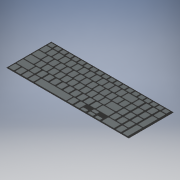
# Autodesk Inventor part: KEYBOARD
Saved by Autodesk Inventor 2017 (Build 210142000, 142)
## iProperties
Created: 2017-02-18
Part Number: KEYBOARD
Material: Generic
Document SubType Name: Modeling
Designer: Ali
Density: 1 g/cm^3
Appearance: Default
Author: Ali
Autodesk Inventor part; units mm, degrees
ref_plane "YZ Plane" through (0, 0, 0) normal (1, 0, 0) x (0, 1, 0)
ref_plane "XZ Plane" through (0, 0, 0) normal (0, 1, 0) x (-1, 0, 0)
ref_plane "XY Plane" through (0, 0, 0) normal (0, 0, 1) x (1, 0, 0)
sketch "Sketch1" plane through (0, 0, 0) normal (0, 1, 0) x (-1, 0, 0)
  line L0 (149.99, -109.99) -> (-149.99, -109.99)
  line L1 (-149.99, -109.99) -> (-149.99, 0)
  line L2 (-149.99, 0) -> (149.99, 0)
  line L3 (149.99, 0) -> (149.99, -109.99)
  dimension "d2" = 299.98
  dimension "d3" = 109.99
  constraints: 8 end point, 2 parallel, 1 horizontal, 1 perpendicular
  measures "d2" distance of L1.end L2.end
  measures "d3" distance of L0.end L1.end
extrude "KEYBOARD BASE" add sketch "Sketch1" along normal blind 0.01
sketch "Sketch2" plane through (0, 0.01, 0) normal (0, 1, 0) x (1, 0, 0)
  line L0 (-146.9909, 107.99) -> (-136.9909, 107.99)
  line L1 (-135.9909, 106.99) -> (-135.9909, 98.99)
  line L2 (-136.9909, 97.99) -> (-146.9909, 97.99)
  line L3 (-147.9909, 98.99) -> (-147.9909, 106.99)
  arc A0 (-146.9909, 107.99) -> (-147.9909, 106.99) centre (-146.9909, 106.99) ccw
  arc A1 (-135.9909, 106.99) -> (-136.9909, 107.99) centre (-136.9909, 106.99) ccw
  arc A2 (-136.9909, 97.99) -> (-135.9909, 98.99) centre (-136.9909, 98.99) ccw
  arc A3 (-147.9909, 98.99) -> (-146.9909, 97.99) centre (-146.9909, 98.99) ccw
  point P0 (0, 0)
  point P1 (-147.9909, 107.99)
  point P2 (-135.9909, 97.99)
  point P3 (-135.9909, 107.99)
  point P4 (-147.9909, 97.99)
  dimension "d9" = 10
  dimension "d10" = 12
  dimension "d150" = 1
  constraints: 8 end point, 8 point on circle, 8 point on line, 8 tangent, 4 centre point, 3 equal radius, 2 parallel, 1 horizontal, 1 perpendicular
  measures "d9" distance of point (-147.991, 97.99) point (-147.991, 107.99)
  measures "d10" distance of point (-147.991, 107.99) point (-135.991, 107.99)
  measures "d150" radius of A0
extrude "ESCAPE BUTTON" add sketch "Sketch2" along normal blind 0.3
pattern_linear "1ST ROW" count 20 spacing 14.75 along (1, 0, 0) of "ESCAPE BUTTON"
sketch "Sketch3" plane through (0, 0.01, 0) normal (0, 1, 0) x (1, 0, 0)
  line L0 (-145.9909, 95.99) -> (-136.4909, 95.99)
  line L1 (-134.4909, 93.99) -> (-134.4909, 80.79)
  line L2 (-136.4909, 78.79) -> (-145.9909, 78.79)
  line L3 (-147.9909, 80.79) -> (-147.9909, 93.99)
  arc A0 (-145.9909, 95.99) -> (-147.9909, 93.99) centre (-145.9909, 93.99) ccw
  arc A1 (-134.4909, 93.99) -> (-136.4909, 95.99) centre (-136.4909, 93.99) ccw
  arc A2 (-136.4909, 78.79) -> (-134.4909, 80.79) centre (-136.4909, 80.79) ccw
  arc A3 (-147.9909, 80.79) -> (-145.9909, 78.79) centre (-145.9909, 80.79) ccw
  point P0 (-147.9909, 95.99)
  point P1 (-134.4909, 78.79)
  point P2 (-134.4909, 95.99)
  point P3 (-147.9909, 78.79)
  dimension "d19" = 13.5
  dimension "d20" = 17.2
  dimension "d151" = 2
  constraints: 8 end point, 8 point on circle, 8 point on line, 8 tangent, 4 centre point, 3 equal radius, 2 parallel, 1 horizontal, 1 perpendicular
  measures "d19" distance of point (-147.991, 95.99) point (-134.491, 95.99)
  measures "d20" distance of point (-147.991, 78.79) point (-147.991, 95.99)
  measures "d151" radius of A0
extrude "2ND ROW" add sketch "Sketch3" along normal blind 0.3
pattern_linear "2ND ROW PATTERN" count 13 spacing 15.5 along (1, 0, 0) of "2ND ROW"
sketch "Sketch6" plane through (0, 0.01, 0) normal (0, 1, 0) x (1, 0, 0)
  line L0 (133.5089, 95.99) -> (143.0089, 95.99)
  line L1 (145.0089, 93.99) -> (145.0089, 80.79)
  line L2 (143.0089, 78.79) -> (133.5089, 78.79)
  line L3 (131.5089, 80.79) -> (131.5089, 93.99)
  arc A0 (133.5089, 95.99) -> (131.5089, 93.99) centre (133.5089, 93.99) ccw
  arc A1 (145.0089, 93.99) -> (143.0089, 95.99) centre (143.0089, 93.99) ccw
  arc A2 (143.0089, 78.79) -> (145.0089, 80.79) centre (143.0089, 80.79) ccw
  arc A3 (131.5089, 80.79) -> (133.5089, 78.79) centre (133.5089, 80.79) ccw
  point P0 (0, 0)
  point P1 (131.5089, 95.99)
  point P2 (145.0089, 78.79)
  point P3 (145.0089, 95.99)
  point P4 (131.5089, 78.79)
  dimension "d52" = 13.5
  dimension "d53" = 17.2
  dimension "d157" = 2
  constraints: 8 end point, 8 point on circle, 8 point on line, 8 tangent, 4 centre point, 3 equal radius, 2 parallel, 1 horizontal, 1 perpendicular
  measures "d52" distance of point (145.009, 78.79) point (131.509, 78.79)
  measures "d53" distance of point (145.009, 95.99) point (145.009, 78.79)
  measures "d157" radius of A0
sketch "Sketch4" plane through (0, 0.01, 0) normal (0, 1, 0) x (1, 0, 0)
  line L0 (55.5091, 95.99) -> (76.5091, 95.99)
  line L1 (78.5091, 93.99) -> (78.5091, 80.79)
  line L2 (76.5091, 78.79) -> (55.5091, 78.79)
  line L3 (53.5091, 80.79) -> (53.5091, 93.99)
  arc A0 (55.5091, 95.99) -> (53.5091, 93.99) centre (55.5091, 93.99) ccw
  arc A1 (78.5091, 93.99) -> (76.5091, 95.99) centre (76.5091, 93.99) ccw
  arc A2 (76.5091, 78.79) -> (78.5091, 80.79) centre (76.5091, 80.79) ccw
  arc A3 (53.5091, 80.79) -> (55.5091, 78.79) centre (55.5091, 80.79) ccw
  point P0 (53.5091, 95.99)
  point P1 (78.5091, 78.79)
  point P2 (78.5091, 95.99)
  point P3 (53.5091, 78.79)
  dimension "d31" = 25
  dimension "d32" = 17.2
  dimension "d156" = 2
  constraints: 8 end point, 8 point on circle, 8 point on line, 8 tangent, 4 centre point, 3 equal radius, 2 parallel, 1 horizontal, 1 perpendicular
  measures "d31" distance of point (78.509, 78.79) point (53.509, 78.79)
  measures "d32" distance of point (78.509, 95.99) point (78.509, 78.79)
  measures "d156" radius of A0
extrude "BACKSPACE BUTTON" add sketch "Sketch4" along normal blind 0.3
sketch "Sketch7" plane through (0, 0.01, 0) normal (0, 1, 0) x (1, 0, 0)
  line L0 (133.5098, 76.99) -> (143.0098, 76.99)
  line L1 (145.0098, 74.99) -> (145.0098, 42.79)
  line L2 (143.0098, 40.79) -> (133.5098, 40.79)
  line L3 (131.5098, 42.79) -> (131.5098, 74.99)
  arc A0 (133.5098, 76.99) -> (131.5098, 74.99) centre (133.5098, 74.99) ccw
  arc A1 (145.0098, 74.99) -> (143.0098, 76.99) centre (143.0098, 74.99) ccw
  arc A2 (143.0098, 40.79) -> (145.0098, 42.79) centre (143.0098, 42.79) ccw
  arc A3 (131.5098, 42.79) -> (133.5098, 40.79) centre (133.5098, 42.79) ccw
  point P0 (0, 0)
  point P1 (131.5098, 76.99)
  point P2 (145.0098, 40.79)
  point P3 (145.0098, 76.99)
  point P4 (131.5098, 40.79)
  dimension "d56" = 13.5
  dimension "d57" = 36.2
  dimension "d158" = 2
  constraints: 8 end point, 8 point on circle, 8 point on line, 8 tangent, 4 centre point, 3 equal radius, 2 parallel, 1 horizontal, 1 perpendicular
  measures "d56" distance of point (145.01, 40.79) point (131.51, 40.79)
  measures "d57" distance of point (145.01, 76.99) point (145.01, 40.79)
  measures "d158" radius of A0
sketch "Sketch5" plane through (0, 0.01, 0) normal (0, 1, 0) x (1, 0, 0)
  line L0 (82.5091, 95.99) -> (92.0091, 95.99)
  line L1 (94.0091, 93.99) -> (94.0091, 80.79)
  line L2 (92.0091, 78.79) -> (82.5091, 78.79)
  line L3 (80.5091, 80.79) -> (80.5091, 93.99)
  arc A0 (82.5091, 95.99) -> (80.5091, 93.99) centre (82.5091, 93.99) ccw
  arc A1 (94.0091, 93.99) -> (92.0091, 95.99) centre (92.0091, 93.99) ccw
  arc A2 (92.0091, 78.79) -> (94.0091, 80.79) centre (92.0091, 80.79) ccw
  arc A3 (80.5091, 80.79) -> (82.5091, 78.79) centre (82.5091, 80.79) ccw
  point P0 (80.5091, 95.99)
  point P1 (94.0091, 78.79)
  point P2 (94.0091, 95.99)
  point P3 (80.5091, 78.79)
  dimension "d152" = 2
  constraints: 8 end point, 8 point on circle, 8 point on line, 8 tangent, 4 centre point, 3 equal radius, 2 parallel, 1 horizontal, 1 perpendicular
  measures "d152" radius of A0
extrude "NUM LOCK BUTTON" add sketch "Sketch5" along normal blind 0.3
pattern_linear "NUMERIC KEYPAD" count 3 spacing 17 along (1, 0, 0) count 4 spacing 19 along (0, 0, 1) of "NUM LOCK BUTTON"
sketch "Sketch9" plane through (0, 0.01, 0) normal (0, 1, 0) x (1, 0, 0)
  line L0 (116.5091, 19.9893) -> (126.0091, 19.9893)
  line L1 (128.0091, 17.9893) -> (128.0091, 4.7893)
  line L2 (126.0091, 2.7893) -> (116.5091, 2.7893)
  line L3 (114.5091, 4.7893) -> (114.5091, 17.9893)
  arc A0 (116.5091, 19.9893) -> (114.5091, 17.9893) centre (116.5091, 17.9893) ccw
  arc A1 (128.0091, 17.9893) -> (126.0091, 19.9893) centre (126.0091, 17.9893) ccw
  arc A2 (126.0091, 2.7893) -> (128.0091, 4.7893) centre (126.0091, 4.7893) ccw
  arc A3 (114.5091, 4.7893) -> (116.5091, 2.7893) centre (116.5091, 4.7893) ccw
  point P0 (0, 0)
  point P1 (114.5091, 19.9893)
  point P2 (128.0091, 2.7893)
  point P3 (128.0091, 19.9893)
  point P4 (114.5091, 2.7893)
  dimension "d160" = 2
  constraints: 8 end point, 8 point on circle, 8 point on line, 8 tangent, 4 centre point, 3 equal radius, 2 parallel, 1 horizontal, 1 perpendicular
  measures "d160" radius of A0
extrude "SUBTRACT BUTTON" add sketch "Sketch6" along normal blind 0.3
sketch "Sketch10" plane through (0, 0.01, 0) normal (0, 1, 0) x (1, 0, 0)
  line L0 (-145.9909, 76.9862) -> (-127.9909, 76.9862)
  line L1 (-125.9909, 74.9862) -> (-125.9909, 61.7862)
  line L2 (-127.9909, 59.7862) -> (-145.9909, 59.7862)
  line L3 (-147.9909, 61.7862) -> (-147.9909, 74.9862)
  arc A0 (-145.9909, 76.9862) -> (-147.9909, 74.9862) centre (-145.9909, 74.9862) ccw
  arc A1 (-125.9909, 74.9862) -> (-127.9909, 76.9862) centre (-127.9909, 74.9862) ccw
  arc A2 (-127.9909, 59.7862) -> (-125.9909, 61.7862) centre (-127.9909, 61.7862) ccw
  arc A3 (-147.9909, 61.7862) -> (-145.9909, 59.7862) centre (-145.9909, 61.7862) ccw
  point P0 (-147.9909, 76.9862)
  point P1 (-125.9909, 59.7862)
  point P2 (-125.9909, 76.9862)
  point P3 (-147.9909, 59.7862)
  dimension "d161" = 2
  constraints: 8 end point, 8 point on circle, 8 point on line, 8 tangent, 4 centre point, 3 equal radius, 2 parallel, 1 horizontal, 1 perpendicular
  measures "d161" radius of A0
extrude "ADD BUTTON" add sketch "Sketch7" along normal blind 0.3
pattern_linear "ENTER BUTTON" count 2 spacing 38 along (0, 0, 1) of "ADD BUTTON"
sketch "Sketch11" plane through (0, 0.01, 0) normal (0, 1, 0) x (1, 0, 0)
  line L0 (-121.9955, 76.9862) -> (-112.4955, 76.9862)
  line L1 (-110.4955, 74.9862) -> (-110.4955, 61.7862)
  line L2 (-112.4955, 59.7862) -> (-121.9955, 59.7862)
  line L3 (-123.9955, 61.7862) -> (-123.9955, 74.9862)
  arc A0 (-121.9955, 76.9862) -> (-123.9955, 74.9862) centre (-121.9955, 74.9862) ccw
  arc A1 (-110.4955, 74.9862) -> (-112.4955, 76.9862) centre (-112.4955, 74.9862) ccw
  arc A2 (-112.4955, 59.7862) -> (-110.4955, 61.7862) centre (-112.4955, 61.7862) ccw
  arc A3 (-123.9955, 61.7862) -> (-121.9955, 59.7862) centre (-121.9955, 61.7862) ccw
  point P0 (0, 0)
  point P1 (-123.9955, 76.9862)
  point P2 (-110.4955, 59.7862)
  point P3 (-110.4955, 76.9862)
  point P4 (-123.9955, 59.7862)
  dimension "d153" = 2
  constraints: 8 end point, 8 point on circle, 8 point on line, 8 tangent, 4 centre point, 3 equal radius, 2 parallel, 1 horizontal, 1 perpendicular
  measures "d153" radius of A0
sketch "Sketch8" plane through (0, 0.01, 0) normal (0, 1, 0) x (1, 0, 0)
  line L0 (82.5091, 19.9863) -> (109.0091, 19.9863)
  line L1 (111.0091, 17.9863) -> (111.0091, 4.7863)
  line L2 (109.0091, 2.7863) -> (82.5091, 2.7863)
  line L3 (80.5091, 4.7863) -> (80.5091, 17.9863)
  arc A0 (82.5091, 19.9863) -> (80.5091, 17.9863) centre (82.5091, 17.9863) ccw
  arc A1 (111.0091, 17.9863) -> (109.0091, 19.9863) centre (109.0091, 17.9863) ccw
  arc A2 (109.0091, 2.7863) -> (111.0091, 4.7863) centre (109.0091, 4.7863) ccw
  arc A3 (80.5091, 4.7863) -> (82.5091, 2.7863) centre (82.5091, 4.7863) ccw
  point P0 (0, 0)
  point P1 (80.5091, 19.9863)
  point P2 (111.0091, 2.7863)
  point P3 (111.0091, 19.9863)
  point P4 (80.5091, 2.7863)
  dimension "d63" = 30.5
  dimension "d64" = 17.2
  dimension "d159" = 2
  constraints: 8 end point, 8 point on circle, 8 point on line, 8 tangent, 4 centre point, 3 equal radius, 2 parallel, 1 horizontal, 1 perpendicular
  measures "d63" distance of point (111.009, 2.786) point (80.509, 2.786)
  measures "d64" distance of point (111.009, 19.986) point (111.009, 2.786)
  measures "d159" radius of A0
extrude "0 BUTTON" add sketch "Sketch8" along normal blind 0.3
sketch "Sketch12" plane through (0, 0.01, 0) normal (0, 1, 0) x (1, 0, 0)
  line L0 (-145.9909, 57.989) -> (-125.9909, 57.989)
  line L1 (-123.9909, 55.989) -> (-123.9909, 42.789)
  line L2 (-125.9909, 40.789) -> (-145.9909, 40.789)
  line L3 (-147.9909, 42.789) -> (-147.9909, 55.989)
  arc A0 (-145.9909, 57.989) -> (-147.9909, 55.989) centre (-145.9909, 55.989) ccw
  arc A1 (-147.9909, 42.789) -> (-145.9909, 40.789) centre (-145.9909, 42.789) ccw
  arc A2 (-125.9909, 40.789) -> (-123.9909, 42.789) centre (-125.9909, 42.789) ccw
  arc A3 (-123.9909, 55.989) -> (-125.9909, 57.989) centre (-125.9909, 55.989) ccw
  point P0 (-147.9909, 57.989)
  point P1 (-123.9909, 40.789)
  point P2 (-123.9909, 57.989)
  point P3 (-147.9909, 40.789)
  dimension "d84" = 24
  dimension "d85" = 17.2
  dimension "d162" = 2
  constraints: 8 end point, 8 point on circle, 8 point on line, 8 tangent, 4 centre point, 3 equal radius, 2 parallel, 1 horizontal, 1 perpendicular
  measures "d84" distance of point (-147.991, 57.989) point (-123.991, 57.989)
  measures "d85" distance of point (-147.991, 40.789) point (-147.991, 57.989)
  measures "d162" radius of A0
extrude "DOT BUTTON" add sketch "Sketch9" along normal blind 0.3
sketch "Sketch13" plane through (0, 0.01, 0) normal (0, 1, 0) x (1, 0, 0)
  line L0 (-119.9959, 57.989) -> (-110.4959, 57.989)
  line L1 (-108.4959, 55.989) -> (-108.4959, 42.789)
  line L2 (-110.4959, 40.789) -> (-119.9959, 40.789)
  line L3 (-121.9959, 42.789) -> (-121.9959, 55.989)
  arc A0 (-119.9959, 57.989) -> (-121.9959, 55.989) centre (-119.9959, 55.989) ccw
  arc A1 (-108.4959, 55.989) -> (-110.4959, 57.989) centre (-110.4959, 55.989) ccw
  arc A2 (-110.4959, 40.789) -> (-108.4959, 42.789) centre (-110.4959, 42.789) ccw
  arc A3 (-121.9959, 42.789) -> (-119.9959, 40.789) centre (-119.9959, 42.789) ccw
  point P0 (0, 0)
  point P1 (-121.9959, 57.989)
  point P2 (-108.4959, 40.789)
  point P3 (-108.4959, 57.989)
  point P4 (-121.9959, 40.789)
  dimension "d154" = 2
  constraints: 8 end point, 8 point on circle, 8 point on line, 8 tangent, 4 centre point, 3 equal radius, 2 parallel, 1 horizontal, 1 perpendicular
  measures "d154" radius of A0
extrude "TAB BUTTON" add sketch "Sketch10" along normal blind 0.3
sketch "Sketch14" plane through (0, 0.01, 0) normal (0, 1, 0) x (1, 0, 0)
  line L0 (52.9992, 57.989) -> (75.9992, 57.989)
  line L1 (77.9992, 55.989) -> (77.9992, 42.789)
  line L2 (75.9992, 40.789) -> (52.9992, 40.789)
  line L3 (50.9992, 42.789) -> (50.9992, 55.989)
  arc A0 (52.9992, 57.989) -> (50.9992, 55.989) centre (52.9992, 55.989) ccw
  arc A1 (77.9992, 55.989) -> (75.9992, 57.989) centre (75.9992, 55.989) ccw
  arc A2 (75.9992, 40.789) -> (77.9992, 42.789) centre (75.9992, 42.789) ccw
  arc A3 (50.9992, 42.789) -> (52.9992, 40.789) centre (52.9992, 42.789) ccw
  point P0 (50.9992, 57.989)
  point P1 (77.9992, 40.789)
  point P2 (77.9992, 57.989)
  point P3 (50.9992, 40.789)
  dimension "d95" = 27
  dimension "d96" = 17.2
  dimension "d163" = 2
  constraints: 8 end point, 8 point on circle, 8 point on line, 8 tangent, 4 centre point, 3 equal radius, 2 parallel, 1 horizontal, 1 perpendicular
  measures "d95" distance of point (77.999, 40.789) point (50.999, 40.789)
  measures "d96" distance of point (77.999, 57.989) point (77.999, 40.789)
  measures "d163" radius of A0
extrude "Q BUTTON" add sketch "Sketch11" along normal blind 0.3
pattern_linear "QWERTY" count 13 spacing 15.7 along (1, 0, 0) of "Q BUTTON"
sketch "Sketch15" plane through (0, 0.01, 0) normal (0, 1, 0) x (1, 0, 0)
  line L0 (-145.9909, 38.9918) -> (-119.9909, 38.9918)
  line L1 (-117.9909, 36.9918) -> (-117.9909, 23.7918)
  line L2 (-119.9909, 21.7918) -> (-145.9909, 21.7918)
  line L3 (-147.9909, 23.7918) -> (-147.9909, 36.9918)
  arc A0 (-145.9909, 38.9918) -> (-147.9909, 36.9918) centre (-145.9909, 36.9918) ccw
  arc A1 (-117.9909, 36.9918) -> (-119.9909, 38.9918) centre (-119.9909, 36.9918) ccw
  arc A2 (-119.9909, 21.7918) -> (-117.9909, 23.7918) centre (-119.9909, 23.7918) ccw
  arc A3 (-147.9909, 23.7918) -> (-145.9909, 21.7918) centre (-145.9909, 23.7918) ccw
  point P0 (-147.9909, 38.9918)
  point P1 (-117.9909, 21.7918)
  point P2 (-117.9909, 38.9918)
  point P3 (-147.9909, 21.7918)
  dimension "d112" = 17.2
  dimension "d113" = 77.5
  dimension "d165" = 2
  dimension "d101" = 30
  dimension "d102" = 17.2
  dimension "d164" = 2
  constraints: 8 end point, 8 point on circle, 8 point on line, 8 tangent, 4 centre point, 3 equal radius, 2 parallel, 1 horizontal, 1 perpendicular
  measures "d101" distance of point (-147.991, 38.992) point (-117.991, 38.992)
  measures "d102" distance of point (-147.991, 21.792) point (-147.991, 38.992)
  measures "d164" radius of A0
extrude "CAPS LOCK" add sketch "Sketch12" along normal blind 0.3
sketch "Sketch16" plane through (0, 0.01, 0) normal (0, 1, 0) x (1, 0, 0)
  line L0 (-113.9901, 38.9918) -> (-104.4901, 38.9918)
  line L1 (-102.4901, 36.9918) -> (-102.4901, 23.7918)
  line L2 (-104.4901, 21.7918) -> (-113.9901, 21.7918)
  line L3 (-115.9901, 23.7918) -> (-115.9901, 36.9918)
  arc A0 (-113.9901, 38.9918) -> (-115.9901, 36.9918) centre (-113.9901, 36.9918) ccw
  arc A1 (-102.4901, 36.9918) -> (-104.4901, 38.9918) centre (-104.4901, 36.9918) ccw
  arc A2 (-104.4901, 21.7918) -> (-102.4901, 23.7918) centre (-104.4901, 23.7918) ccw
  arc A3 (-115.9901, 23.7918) -> (-113.9901, 21.7918) centre (-113.9901, 23.7918) ccw
  point P0 (0, 0)
  point P1 (-115.9901, 38.9918)
  point P2 (-102.4901, 21.7918)
  point P3 (-102.4901, 38.9918)
  point P4 (-115.9901, 21.7918)
  dimension "d155" = 2
  constraints: 8 end point, 8 point on circle, 8 point on line, 8 tangent, 4 centre point, 3 equal radius, 2 parallel, 1 horizontal, 1 perpendicular
  measures "d155" radius of A0
extrude "A BUTTON" add sketch "Sketch13" along normal blind 0.3
pattern_linear "ASDFGH" count 11 spacing 15.75 along (1, 0, 0) of "A BUTTON"
sketch "Sketch17" plane through (0, 0.01, 0) normal (0, 1, 0) x (1, 0, 0)
  line L0 (-81.9901, 19.9885) -> (-8.4901, 19.9885)
  line L1 (-6.4901, 17.9885) -> (-6.4901, 4.7885)
  line L2 (-8.4901, 2.7885) -> (-81.9901, 2.7885)
  line L3 (-83.9901, 4.7885) -> (-83.9901, 17.9885)
  arc A0 (-81.9901, 19.9885) -> (-83.9901, 17.9885) centre (-81.9901, 17.9885) ccw
  arc A1 (-6.4901, 17.9885) -> (-8.4901, 19.9885) centre (-8.4901, 17.9885) ccw
  arc A2 (-8.4901, 2.7885) -> (-6.4901, 4.7885) centre (-8.4901, 4.7885) ccw
  arc A3 (-83.9901, 4.7885) -> (-81.9901, 2.7885) centre (-81.9901, 4.7885) ccw
  point P0 (-83.9901, 19.9885)
  point P1 (-6.4901, 2.7885)
  point P2 (-6.4901, 19.9885)
  point P3 (-83.9901, 2.7885)
  dimension "d112" = 17.2
  dimension "d113" = 77.5
  dimension "d165" = 2
  constraints: 8 end point, 8 point on circle, 8 point on line, 8 tangent, 4 centre point, 3 equal radius, 2 parallel, 1 horizontal, 1 perpendicular
  measures "d112" distance of point (-6.49, 19.989) point (-6.49, 2.789)
  measures "d113" distance of point (-6.49, 2.789) point (-83.99, 2.789)
  measures "d165" radius of A0
extrude "ENTER BUTTON 1" add sketch "Sketch14" along normal blind 0.3
sketch "Sketch18" plane through (0, 0.01, 0) normal (0, 1, 0) x (1, 0, 0)
  line L0 (75.9992, 38.9909) -> (49.9992, 38.9909)
  line L1 (47.9992, 36.9909) -> (47.9992, 23.7909)
  line L2 (49.9992, 21.7909) -> (75.9992, 21.7909)
  line L3 (77.9992, 23.7909) -> (77.9992, 36.9909)
  arc A0 (49.9992, 38.9909) -> (47.9992, 36.9909) centre (49.9992, 36.9909) ccw
  arc A1 (77.9992, 36.9909) -> (75.9992, 38.9909) centre (75.9992, 36.9909) ccw
  arc A2 (75.9992, 21.7909) -> (77.9992, 23.7909) centre (75.9992, 23.7909) ccw
  arc A3 (47.9992, 23.7909) -> (49.9992, 21.7909) centre (49.9992, 23.7909) ccw
  point P0 (77.9992, 38.9909)
  point P1 (47.9992, 21.7909)
  point P2 (47.9992, 38.9909)
  point P3 (77.9992, 21.7909)
  dimension "d166" = 2
  constraints: 8 end point, 8 point on circle, 8 point on line, 8 tangent, 4 centre point, 3 equal radius, 2 parallel, 1 horizontal, 1 perpendicular
  measures "d166" radius of A0
extrude "LEFT SHIFT" add sketch "Sketch15" along normal blind 0.3
sketch "Sketch19" plane through (0, 0.01, 0) normal (0, 1, 0) x (1, 0, 0)
  line L0 (-145.9909, 19.9917) -> (-136.4909, 19.9917)
  line L1 (-134.4909, 17.9917) -> (-134.4909, 4.7917)
  line L2 (-136.4909, 2.7917) -> (-145.9909, 2.7917)
  line L3 (-147.9909, 4.7917) -> (-147.9909, 17.9917)
  arc A0 (-145.9909, 19.9917) -> (-147.9909, 17.9917) centre (-145.9909, 17.9917) ccw
  arc A1 (-134.4909, 17.9917) -> (-136.4909, 19.9917) centre (-136.4909, 17.9917) ccw
  arc A2 (-136.4909, 2.7917) -> (-134.4909, 4.7917) centre (-136.4909, 4.7917) ccw
  arc A3 (-147.9909, 4.7917) -> (-145.9909, 2.7917) centre (-145.9909, 4.7917) ccw
  point P0 (0, 0)
  point P1 (-147.9909, 19.9917)
  point P2 (-134.4909, 2.7917)
  point P3 (-134.4909, 19.9917)
  point P4 (-147.9909, 2.7917)
  dimension "d167" = 2
  constraints: 8 end point, 8 point on circle, 8 point on line, 8 tangent, 4 centre point, 3 equal radius, 2 parallel, 1 horizontal, 1 perpendicular
  measures "d167" radius of A0
extrude "Z BUTTON" add sketch "Sketch16" along normal blind 0.3
pattern_linear "ZXCVBN" count 10 spacing 16.5 along (1, 0, 0) of "Z BUTTON"
sketch "Sketch20" plane through (0, 0.01, 0) normal (0, 1, 0) x (1, 0, 0)
  line L0 (-2.4885, 19.9885) -> (7.0115, 19.9885)
  line L1 (9.0115, 17.9885) -> (9.0115, 4.7885)
  line L2 (7.0115, 2.7885) -> (-2.4885, 2.7885)
  line L3 (-4.4885, 4.7885) -> (-4.4885, 17.9885)
  arc A0 (-2.4885, 19.9885) -> (-4.4885, 17.9885) centre (-2.4885, 17.9885) ccw
  arc A1 (9.0115, 17.9885) -> (7.0115, 19.9885) centre (7.0115, 17.9885) ccw
  arc A2 (7.0115, 2.7885) -> (9.0115, 4.7885) centre (7.0115, 4.7885) ccw
  arc A3 (-4.4885, 4.7885) -> (-2.4885, 2.7885) centre (-2.4885, 4.7885) ccw
  point P0 (-4.4885, 19.9885)
  point P1 (9.0115, 2.7885)
  point P2 (9.0115, 19.9885)
  point P3 (-4.4885, 2.7885)
  dimension "d168" = 2
  constraints: 8 end point, 8 point on circle, 8 point on line, 8 tangent, 4 centre point, 3 equal radius, 2 parallel, 1 horizontal, 1 perpendicular
  measures "d168" radius of A0
extrude "SPACE BAR" add sketch "Sketch17" along normal blind 0.3
sketch "Sketch21" plane through (0, 0.01, 0) normal (0, 1, 0) x (1, 0, 0)
  line L0 (30.0093, 2.7885) -> (39.5093, 2.7885)
  line L1 (41.5093, 4.7885) -> (41.5093, 8.2885)
  line L2 (39.5093, 10.2885) -> (30.0093, 10.2885)
  line L3 (28.0093, 8.2885) -> (28.0093, 4.7885)
  arc A0 (30.0093, 10.2885) -> (28.0093, 8.2885) centre (30.0093, 8.2885) ccw
  arc A1 (41.5093, 8.2885) -> (39.5093, 10.2885) centre (39.5093, 8.2885) ccw
  arc A2 (39.5093, 2.7885) -> (41.5093, 4.7885) centre (39.5093, 4.7885) ccw
  arc A3 (28.0093, 4.7885) -> (30.0093, 2.7885) centre (30.0093, 4.7885) ccw
  point P0 (28.0093, 2.7885)
  point P1 (41.5093, 10.2885)
  point P2 (41.5093, 2.7885)
  point P3 (28.0093, 10.2885)
  dimension "d136" = 13.5
  dimension "d137" = 7.5
  dimension "d170" = 2
  constraints: 8 end point, 8 point on circle, 8 point on line, 8 tangent, 4 centre point, 3 equal radius, 2 parallel, 1 horizontal, 1 perpendicular
  measures "d136" distance of point (28.009, 2.789) point (41.509, 2.789)
  measures "d137" distance of point (28.009, 10.289) point (28.009, 2.789)
  measures "d170" radius of A0
extrude "RIGHT SHIFT" add sketch "Sketch18" along normal blind 0.3
sketch "Sketch22" plane through (0, 0.01, 0) normal (0, 1, 0) x (1, 0, 0)
  line L0 (47.5093, 12.0849) -> (57.0093, 12.0849)
  line L1 (59.0093, 14.0849) -> (59.0093, 17.5849)
  line L2 (57.0093, 19.5849) -> (47.5093, 19.5849)
  line L3 (45.5093, 17.5849) -> (45.5093, 14.0849)
  arc A0 (47.5093, 19.5849) -> (45.5093, 17.5849) centre (47.5093, 17.5849) ccw
  arc A1 (59.0093, 17.5849) -> (57.0093, 19.5849) centre (57.0093, 17.5849) ccw
  arc A2 (57.0093, 12.0849) -> (59.0093, 14.0849) centre (57.0093, 14.0849) ccw
  arc A3 (45.5093, 14.0849) -> (47.5093, 12.0849) centre (47.5093, 14.0849) ccw
  point P0 (0, 0)
  point P1 (45.5093, 12.0849)
  point P2 (59.0093, 19.5849)
  point P3 (59.0093, 12.0849)
  point P4 (45.5093, 19.5849)
  dimension "d169" = 2
  constraints: 8 end point, 8 point on circle, 8 point on line, 8 tangent, 4 centre point, 3 equal radius, 2 parallel, 1 horizontal, 1 perpendicular
  measures "d169" radius of A0
extrude "CTRL BUTTON" add sketch "Sketch19" along normal blind 0.3
pattern_linear "FN/WIN/ALT" count 4 spacing 16 along (1, 0, 0) of "CTRL BUTTON"
extrude "ALT BUTTON" add sketch "Sketch20" along normal blind 0.3
pattern_linear "CTRL RIGHT" count 2 spacing 17 along (1, 0, 0) of "ALT BUTTON"
extrude "LEFT ARROW KEY" add sketch "Sketch21" along normal blind 0.3
pattern_linear "ARROW KEYS" count 3 spacing 17.5 along (1, 0, 0) of "LEFT ARROW KEY"
extrude "UP ARROW KEY" add sketch "Sketch22" along normal blind 0.3
body "Solid1"
